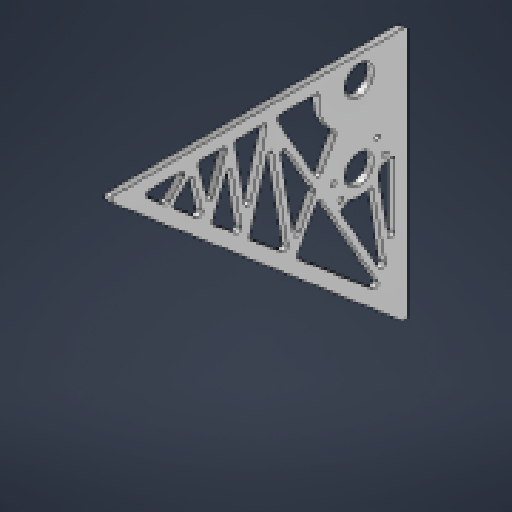
# Autodesk Inventor part: PLATE,GUSSET
Saved by Autodesk Inventor 2026.1 (Build 301233020, 233B)
## iProperties
Created: 2026-03-19
Part Number: PLATE,GUSSET
Material: Aluminum 6061
Document SubType Name: Sheet Metal
Designer: Owen L
Mass: 385.963 g
Surface Area: 536.634 cm^2
Volume: 142.949 cm^3
Density: 2.7 g/cm^3
Sheet Metal Rule: Default
Appearance: Aluminum - Flat
Author: Owen L
Autodesk Inventor part; units mm, degrees
ref_plane "YZ Plane" through (0, 0, 0) normal (1, 0, 0) x (0, 1, 0)
ref_plane "XZ Plane" through (0, 0, 0) normal (0, 1, 0) x (-1, 0, 0)
ref_plane "XY Plane" through (0, 0, 0) normal (0, 0, 1) x (1, 0, 0)
sketch "Sketch1" plane through (0, 0, 0) normal (1, 0, 0) x (0, 1, 0)
  line L0 (0, 0) -> (-254, 0)
  line L1 (0, 349.25) -> (0, 0)
  circle A0 centre (-19.05, 47.625) radius 14.2875
  line L2 (-254, 0) -> (-254, 34.925)
  line L3 (0, 349.25) -> (-44.45, 349.25)
  circle A1 centre (-19.05, 314.325) radius 14.2875
  line L4 (-254, 34.925) -> (-92.075, 34.925)
  line L5 (-92.075, 34.925) -> (-44.45, 74.8871)
  line L6 (-44.45, 74.8871) -> (-44.45, 349.25)
  dimension "d2" = 254
  dimension "d3" = 349.25
  dimension "d5" = 47.625
  dimension "d6" = 19.05
  dimension "d7" = 28.575
  dimension "d45" = 34.925
  dimension "d47" = 44.45
  dimension "d50" = 266.7
  dimension "d51" = 130
  dimension "d52" = 161.925
  measures "d2" distance of L0.start L0.end
  measures "d3" distance of L1.start L0.start
  measures "d5" distance from line of L0 A0.centre
  measures "d6" distance from line of L1 A0.centre
  measures "d7" diameter of A0
  measures "d45" distance of L0.end L2.end
  measures "d47" distance of L1.start L3.end
  measures "d50" distance of A0.centre A1.centre
  measures "d51" angle of L6 L5
  measures "d52" distance of L2.end L4.end
extrude "Plate1" add sketch "Sketch1" along normal blind 6.35
equation "\"d4\" = Thickness"
equation "\"BendRadius\" = Thickness"
equation "\"BendReliefWidth\" = Thickness"
equation "\"BendReliefDepth\" = 0.5 * Thickness"
equation "\"CornerReliefSize\" = 4 * Thickness"
equation "\"MinimumRemnant\" = 2 * Thickness"
equation "\"TransitionRadius\" = BendRadius"
equation "\"JacobiRadiusSize\" = BendRadius"
equation "\"GapSize\" = Thickness"
equation "\"Thickness\" = 6.35"
body "Solid1"
